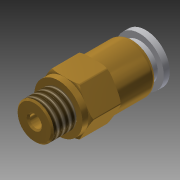
# Autodesk Inventor part: pc4_m10
Saved by Autodesk Inventor 2013 (Build 170138000, 138)
## iProperties
Created: 2015-02-20
Part Number: pc4_m10
Material: 一般
Document SubType Name: Modeling
Designer: Noa Izumi
Density: 1 g/cm^3
Author: Noa Izumi
Autodesk Inventor part; units mm, degrees
ref_plane "YZ Plane" through (0, 0, 0) normal (1, 0, 0) x (0, 1, 0)
ref_plane "XZ Plane" through (0, 0, 0) normal (0, 1, 0) x (-1, 0, 0)
ref_plane "XY Plane" through (0, 0, 0) normal (0, 0, 1) x (1, 0, 0)
sketch "草圖1" plane through (0, 0, 0) normal (0, 1, 0) x (-1, 0, 0)
  circle A0 centre (0, 0) radius 4
  dimension "d0" = 8
  constraints: 1 centre point, 1 coincident
  measures "d0" diameter of A0
extrude "擠出1" add sketch "草圖1" along normal blind 1
sketch "草圖2" plane through (0, 1, 0) normal (0, 1, 0) x (1, 0, 0)
  circle A0 centre (0, 0) radius 4 projected
  line L0 (2.3094, 4) -> (4.6188, 0)
  line L1 (4.6188, 0) -> (2.3094, -4)
  line L2 (2.3094, -4) -> (-2.3094, -4)
  line L3 (-2.3094, -4) -> (-4.6188, 0)
  line L4 (-4.6188, 0) -> (-2.3094, 4)
  line L5 (-2.3094, 4) -> (2.3094, 4)
  point P0 (0, 4)
  constraints: 12 end point, 1 coincident, 1 midpoint, 1 vertical alignment, 14 other
extrude "擠出2" add sketch "草圖2" along normal blind 5
sketch "草圖3" plane through (0, 6, 0) normal (0, 1, 0) x (1, 0, 0)
  circle A0 centre (0, 0) radius 4
  dimension "d49" = 8
  constraints: 1 centre point, 1 coincident
  measures "d49" diameter of A0
extrude "擠出3" add sketch "草圖3" along normal blind 6.5
fillet "圓角1" radius 1 1 edges at (-4, 12.5, 0)
sketch "草圖4" plane through (0, 12.5, 0) normal (0, 1, 0) x (1, 0, 0)
  circle A0 centre (0, 0) radius 3 projected
  circle A1 centre (0, 0) radius 3
  constraints: 1 centre point, 1 coincident, 1 concentric
extrude "擠出4" add sketch "草圖4" along normal blind 1
sketch "草圖5" plane through (0, 13.5, 0) normal (0, 1, 0) x (1, 0, 0)
  circle A0 centre (0, 0) radius 3 projected
  circle A1 centre (0, 0) radius 4
  dimension "d11" = 8
  constraints: 1 centre point, 1 coincident
  measures "d11" diameter of A1
extrude "擠出5" add sketch "草圖5" along normal blind 1 contours A0 | A1
fillet "圓角2" radius 0.25 6 edges at (4.6188, 3.5, 0) (2.3094, 3.5, 4) (2.3094, 3.5, -4) (-2.3094, 3.5, -4) (-4.6188, 3.5, 0) (-2.3094, 3.5, 4)
sketch "草圖9" plane through (0, 0, 0) normal (0, 0, 1) x (1, 0, 0)
  line L0 (-4.75, 6) -> (-4, 6)
  line L1 (-4.75, 1) -> (-4, 1)
  line L2 (-4.75, 6) -> (-4.75, 5.5)
  line L3 (-4.75, 1) -> (-4.75, 1.5)
  arc A0 (-4, 6) -> (-4.75, 5.5) centre (-4, 5.1875) ccw
  arc A1 (-4.75, 1.5) -> (-4, 1) centre (-4, 1.8125) ccw
  line L4 (0, 0) -> (0, 9)
  dimension "d39" = 1
  dimension "d40" = 5
  dimension "d41" = 4
  dimension "d42" = 4
  dimension "d43" = 0.75
  dimension "d44" = 0.75
  dimension "d45" = 0.5
  dimension "d46" = 0.5
  constraints: 10 end point, 4 point on circle, 2 centre point, 2 parallel, 2 tangent, 1 collinear, 1 horizontal, 1 perpendicular
  measures "d39" distance from line of L4.start L1
  measures "d40" distance between parallel lines of L1 L0
  measures "d41" horizontal distance of L4.start L1.end
  measures "d42" horizontal distance of L4.start L0.end
  measures "d43" distance of L0.start L0.end
  measures "d44" distance of L1.start L1.end
  measures "d45" distance of L0.start L2.end
  measures "d46" distance of L1.start L3.end
revolve "迴轉1" cut sketch "草圖9" angle 360 about axis through (0, 0, 0) along (0, 1, 0)
sketch "草圖10" plane through (0, 0, 0) normal (0, -1, 0) x (1, 0, 0)
  circle A0 centre (0, 0) radius 4 projected
  circle A1 centre (0, 0) radius 3
  dimension "d54" = 6
  constraints: 1 centre point, 1 coincident
  measures "d54" diameter of A1
extrude "擠出6" add sketch "草圖10" along normal blind 4 contours A1
thread "螺紋2" size "M6x1" class "6g" standard "ANSI Metric M Profile" full length
sketch "草圖11" plane through (0, 14.5, 0) normal (0, 1, 0) x (1, 0, 0)
  circle A0 centre (0, 0) radius 4 projected
  constraints: 1 coincident
hole "孔4" at (0, 14.5, 0) direction (0, -1, 0) diameter 2 end through all counterbore diameter 4 counterbore depth 10
chamfer "倒角1" distance 0.25 angle 45 2 edges at (-3, -4, 0) (0, -4, -1)
